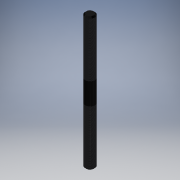
# Autodesk Inventor part: Randverbinder1
Saved by Autodesk Inventor 2019 (Build 230136000, 136)
## iProperties
Created: 2016-08-17
Part Number: Randverbinder1
Material: PC/ABS-Kunststoff
Description: Bodenplatte
Document SubType Name: Modeling
Designer: Gruber
Mass: 1097.46 g
Surface Area: 1699.95 cm^2
Volume: 1097.46 cm^3
Density: 0.357273 g/cm^3
Appearance: Glänzend - Schwarz
AIMD_ORIGIN: ENG-010834
Title: Bodenplatte
Author: Gruber
Autodesk Inventor part; units mm, degrees
ref_plane "YZ Plane" through (0, 0, 0) normal (1, 0, 0) x (0, 1, 0)
ref_plane "XZ Plane" through (0, 0, 0) normal (0, 1, 0) x (-1, 0, 0)
ref_plane "XY Plane" through (0, 0, 0) normal (0, 0, 1) x (1, 0, 0)
sketch "Skizze12" plane through (0, 0, 0) normal (0, 0, 1) x (1, 0, 0)
  circle A0 centre (0, 0) radius 20
  dimension "d77" = 40
  constraints: 1 centre point, 1 coincident
  measures "d77" diameter of A0
extrude "Extrusion11" add sketch "Skizze12" along normal blind 550
chamfer "Fase1" distance 5 angle 45 2 edges at (-20, 0, 0) (-20, 0, 550)
thread "Gewinde2" size "M40x3" class "6g" standard "ANSI Metric M Profile" length 225
thread "Gewinde3" size "M40x3" class "6g" standard "ANSI Metric M Profile" length 225
